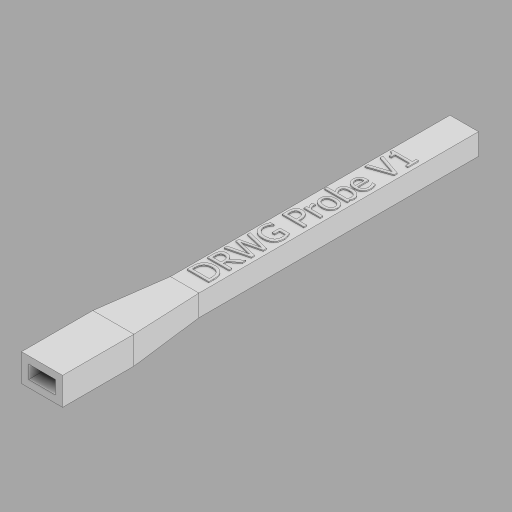
# Autodesk Inventor part: DRWG_ProbeAntenna_V1
Saved by Autodesk Inventor 2023 (Build 270158000, 158)
## iProperties
Created: 2024-10-22
Part Number: DRWG_ProbeAntenna_V1
Material: Generisch
Document SubType Name: Modeling
Designer: Nils Bade
Density: 1 g/cm^3
Appearance: Vorgabe
Author: Nils Bade
Autodesk Inventor part; units mm, degrees
ref_plane "YZ Plane" through (0, 0, 0) normal (1, 0, 0) x (0, 1, 0)
ref_plane "XZ Plane" through (0, 0, 0) normal (0, 1, 0) x (-1, 0, 0)
ref_plane "XY Plane" through (0, 0, 0) normal (0, 0, 1) x (1, 0, 0)
sketch "Skizze1" plane through (0, 0, 0) normal (0, 0, 1) x (1, 0, 0)
  line L0 (-1, 0.5) -> (1, 0.5)
  line L1 (1, 0.5) -> (1, -0.5)
  line L2 (1, -0.5) -> (-1, -0.5)
  line L3 (-1, -0.5) -> (-1, 0.5)
  line L4 (-1, 0.5) -> (1, -0.5) construction
  line L5 (1, 0.5) -> (-1, -0.5) construction
  line L6 (-0.35, 0.5) -> (0.35, 0.5)
  line L7 (0.35, 0.5) -> (0.35, 0.275)
  line L8 (0.35, 0.275) -> (-0.35, 0.275)
  line L9 (-0.35, 0.275) -> (-0.35, 0.5)
  line L10 (0, -2.1) -> (0, 2.1) construction
  line L11 (-2.8, 0) -> (2.8, 0) construction
  line L12 (-0.35, -0.5) -> (0.35, -0.5)
  line L13 (0.35, -0.5) -> (0.35, -0.275)
  line L14 (0.35, -0.275) -> (-0.35, -0.275)
  line L15 (-0.35, -0.275) -> (-0.35, -0.5)
  line L16 (2, 1.5) -> (-2, 1.5)
  line L17 (-2, 1.5) -> (-2, -1.5)
  line L18 (-2, -1.5) -> (2, -1.5)
  line L19 (2, -1.5) -> (2, 1.5)
  point P0 (0, 0)
  point P1 (0, 0.5)
  point P2 (0, 0.5)
  point P3 (0, -0.5)
  point P4 (0, -0.5)
  dimension "d0" = 2
  dimension "d1" = 1
  dimension "d2" = 0.7
  dimension "d3" = 0.55
  dimension "d4" = 1
  constraints: 36 end point, 6 parallel, 6 symmetric about line, 4 midpoint, 3 perpendicular, 3 point on line, 2 horizontal, 3 other
  measures "d0" distance of L1.end L2.end
  measures "d1" distance of L0.end L1.end
  measures "d2" distance of L7.end L8.end
  measures "d3" distance between parallel lines of L8 L14
  measures "d4" distance between parallel lines of L0 L16
extrude "Extrusion1" add sketch "Skizze1" along normal blind 50 contours L0 L7 L8 L9 | L15 L14 L13 L2 | L19 L18 L17 L16
sketch "Skizze2" plane through (0, 0, 0) normal (0, 0, 1) x (1, 0, 0)
  line L0 (1.8795, 0.94) -> (-1.8795, 0.94)
  line L1 (-1.8795, 0.94) -> (-1.8795, -0.94)
  line L2 (-1.8795, -0.94) -> (1.8795, -0.94)
  line L3 (1.8795, -0.94) -> (1.8795, 0.94)
  line L4 (1.8795, 0.94) -> (-1.8795, -0.94) construction
  line L5 (-1.8795, 0.94) -> (1.8795, -0.94) construction
  line L6 (-2.8795, 1.94) -> (2.8795, 1.94)
  line L7 (2.8795, 1.94) -> (2.8795, -1.94)
  line L8 (2.8795, -1.94) -> (-2.8795, -1.94)
  line L9 (-2.8795, -1.94) -> (-2.8795, 1.94)
  point P0 (0, 0)
  dimension "d7" = 3.759
  dimension "d8" = 1.88
  dimension "d9" = 1
  constraints: 20 end point, 4 parallel, 2 midpoint, 2 perpendicular, 1 horizontal, 3 other
  measures "d7" distance of L1.end L2.end
  measures "d8" distance of L0.end L1.end
  measures "d9" distance between parallel lines of L0 L6
extrude "Extrusion2" add sketch "Skizze2" along normal blind 10 from surface at 50
chamfer "Fase1-Taper" distance 0.879 distance2 20 1 edges at (-1, 0, 50) measured on face at (-1.5, 0, 50)
chamfer "Fase2-Taper" distance 0.879 distance2 20 1 edges at (1, 0, 50) measured on face at (1.5, 0, 50)
chamfer "Fase3-Taper" distance 0.44 distance2 20 4 edges at (1.4395, -0.5, 50) (0.675, -0.5, 50) (-0.675, -0.5, 50) (-1.4395, -0.5, 50) measured on face at (1.4395, -0.6, 50) measured on face at (-0.675, -0.6, 50) measured on face at (0.675, -0.6, 50) measured on face at (-1.4395, -0.6, 50)
chamfer "Fase4-Taper" distance 0.44 distance2 20 2 edges at (-1.4395, 0.5, 50) (-0.675, 0.5, 50) measured on face at (-1.4395, 0.6, 50) measured on face at (-0.675, 0.6, 50)
chamfer "Fase5-Taper" distance 0.44 distance2 20 2 edges at (0.675, 0.5, 50) (1.4395, 0.5, 50) measured on face at (0.675, 0.6, 50) measured on face at (1.4395, 0.6, 50)
chamfer "Fase7-Taper" distance 0.665 distance2 20 1 edges at (0, 0.275, 50) measured on face at (0, 0.775, 50)
chamfer "Fase8-Taper" distance 0.665 distance2 20 1 edges at (0, -0.275, 50) measured on face at (0, -0.775, 50)
chamfer "Fase9" distance 0.8 angle 45 4 edges at (0, 1.5, 0) (2, 0, 0) (0, -1.5, 0) (-2, 0, 0)
chamfer "Fase10" [suppressed]
chamfer "Fase11" distance 0.44 distance2 10 1 edges at (0, 1.5, 50) measured on face at (0, 1.6, 50)
chamfer "Fase12" distance 0.44 distance2 10 1 edges at (0, -1.5, 50) measured on face at (0, -1.6, 50)
chamfer "Fase13" distance 0.879 distance2 10 3 edges at (2, -1.72, 50) (2, 0, 50) (2, 1.72, 50) measured on face at (2.5, 1.72, 50) measured on face at (2.5, 0, 50) measured on face at (2.5, -1.72, 50)
chamfer "Fase14" distance 0.879 distance2 10 3 edges at (-2, -1.72, 50) (-2, 0, 50) (-2, 1.72, 50) measured on face at (-2.5, 0, 50) measured on face at (-2.5, -1.72, 50) measured on face at (-2.5, 1.72, 50)
ref_plane "CutSimEnde" through (0, 0, 10) normal (0, 0, -1) x (-1, 0, 0)
feature "Trennen1" [suppressed]
sketch "Skizze3" plane through (-2, 1.5, 0.8) normal (0, 1, 0) x (1, 0, 0)
  line L0 (0.2777, -37.5866) -> (0.2777, -7.5364) construction
  line L1 (0.2777, -7.5364) -> (3.5258, -7.5364) construction
  line L2 (3.5258, -7.5364) -> (3.5258, -37.5866) construction
  line L3 (3.5258, -37.5866) -> (0.2777, -37.5866) construction
  spline S0 degree 2 poles (1.9401, -34.8746) (2.3575, -34.8746) (3.0293, -35.213) (3.2171, -35.497) knots 0 0 0 1 2 2 2
  spline S1 degree 2 poles (3.2171, -35.497) (3.3628, -35.7292) (3.4616, -36.2059) (3.4616, -36.5764) knots 0 0 0 1 2 2 2
  line L4 (3.4616, -36.5764) -> (3.4616, -37.2779)
  line L5 (3.4616, -37.2779) -> (0.4136, -37.2779)
  line L6 (0.4136, -37.2779) -> (0.4136, -36.5838)
  spline S2 degree 2 poles (0.4136, -36.5838) (0.4136, -36.154) (0.542, -35.665) (0.6557, -35.4921) knots 0 0 0 1 2 2 2
  spline S3 degree 2 poles (0.6557, -35.4921) (0.8508, -35.1981) (1.4955, -34.8746) (1.9401, -34.8746) knots 0 0 0 1 2 2 2
  spline S4 degree 2 poles (1.9351, -35.2969) (1.5844, -35.2969) (1.0879, -35.5291) (0.9471, -35.7588) knots 0 0 0 1 2 2 2
  spline S5 degree 2 poles (0.9471, -35.7588) (0.8508, -35.9219) (0.7643, -36.2899) (0.7643, -36.5641) knots 0 0 0 1 2 2 2
  line L7 (0.7643, -36.5641) -> (0.7643, -36.8728)
  line L8 (0.7643, -36.8728) -> (3.1109, -36.8728)
  line L9 (3.1109, -36.8728) -> (3.1109, -36.5641)
  spline S6 degree 2 poles (3.1109, -36.5641) (3.1109, -36.2948) (3.0244, -35.8873) (2.9083, -35.7218) knots 0 0 0 1 2 2 2
  spline S7 degree 2 poles (2.9083, -35.7218) (2.765, -35.5094) (2.2908, -35.2969) (1.9351, -35.2969) knots 0 0 0 1 2 2 2
  line L10 (3.4616, -32.076) -> (3.4616, -32.6022)
  line L11 (3.4616, -32.6022) -> (2.2488, -33.5655)
  line L12 (2.2488, -33.5655) -> (2.2488, -34.0298)
  line L13 (2.2488, -34.0298) -> (3.4616, -34.0298)
  line L14 (3.4616, -34.0298) -> (3.4616, -34.4349)
  line L15 (3.4616, -34.4349) -> (0.4136, -34.4349)
  line L16 (0.4136, -34.4349) -> (0.4136, -33.6494)
  spline S8 degree 2 poles (0.4136, -33.6494) (0.4136, -33.3876) (0.4704, -33.0344) (0.5741, -32.8739) knots 0 0 0 1 2 2 2
  spline S9 degree 2 poles (0.5741, -32.8739) (0.6779, -32.7133) (1.0015, -32.5281) (1.241, -32.5281) knots 0 0 0 1 2 2 2
  spline S10 degree 2 poles (1.241, -32.5281) (1.5745, -32.5281) (2.0265, -32.8689) (2.1352, -33.1604) knots 0 0 0 1 2 2 2
  line L17 (2.1352, -33.1604) -> (3.4616, -32.076)
  spline S11 degree 2 poles (1.2732, -32.9504) (1.1398, -32.9504) (0.9348, -33.0443) (0.8681, -33.1431) knots 0 0 0 1 2 2 2
  spline S12 degree 2 poles (0.8681, -33.1431) (0.8113, -33.2295) (0.7643, -33.4593) (0.7643, -33.6272) knots 0 0 0 1 2 2 2
  line L18 (0.7643, -33.6272) -> (0.7643, -34.0298)
  line L19 (0.7643, -34.0298) -> (1.9104, -34.0298)
  line L20 (1.9104, -34.0298) -> (1.9104, -33.6741)
  spline S13 degree 2 poles (1.9104, -33.6741) (1.9104, -33.4988) (1.8487, -33.2197) (1.7523, -33.1233) knots 0 0 0 1 2 2 2
  spline S14 degree 2 poles (1.7523, -33.1233) (1.6684, -33.0344) (1.4312, -32.9504) (1.2732, -32.9504) knots 0 0 0 1 2 2 2
  line L21 (0.4136, -28.4179) -> (3.4616, -29.1837)
  line L22 (3.4616, -29.1837) -> (3.4616, -29.6381)
  line L23 (3.4616, -29.6381) -> (0.9323, -30.2581)
  line L24 (0.9323, -30.2581) -> (3.4616, -30.8608)
  line L25 (3.4616, -30.8608) -> (3.4616, -31.3103)
  line L26 (3.4616, -31.3103) -> (0.4136, -32.0884)
  line L27 (0.4136, -32.0884) -> (0.4136, -31.671)
  line L28 (0.4136, -31.671) -> (2.9404, -31.0584)
  line L29 (2.9404, -31.0584) -> (0.4136, -30.4508)
  line L30 (0.4136, -30.4508) -> (0.4136, -30.0383)
  line L31 (0.4136, -30.0383) -> (2.9701, -29.4257)
  line L32 (2.9701, -29.4257) -> (0.4136, -28.8156)
  line L33 (0.4136, -28.8156) -> (0.4136, -28.4179)
  spline S15 degree 2 poles (3.5209, -26.7779) (3.5209, -27.1014) (3.3233, -27.6374) (3.1232, -27.8301) knots 0 0 0 1 2 2 2
  spline S16 degree 2 poles (3.1232, -27.8301) (2.9207, -28.0227) (2.3229, -28.2278) (1.9351, -28.2278) knots 0 0 0 1 2 2 2
  spline S17 degree 2 poles (1.9351, -28.2278) (1.5671, -28.2278) (0.9842, -28.0203) (0.7767, -27.8276) knots 0 0 0 1 2 2 2
  spline S18 degree 2 poles (0.7767, -27.8276) (0.5766, -27.6424) (0.3593, -27.099) (0.3593, -26.7754) knots 0 0 0 1 2 2 2
  spline S19 degree 2 poles (0.3593, -26.7754) (0.3593, -26.6198) (0.4037, -26.3382) (0.4432, -26.2098) knots 0 0 0 1 2 2 2
  spline S20 degree 2 poles (0.4432, -26.2098) (0.4729, -26.106) (0.5816, -25.8541) (0.6211, -25.7775) knots 0 0 0 1 2 2 2
  line L34 (0.6211, -25.7775) -> (1.1101, -25.7775)
  line L35 (1.1101, -25.7775) -> (1.1101, -25.8121)
  spline S21 degree 2 poles (1.1101, -25.8121) (1.0434, -25.8887) (0.9224, -26.0492) (0.8533, -26.1974) knots 0 0 0 1 2 2 2
  spline S22 degree 2 poles (0.8533, -26.1974) (0.7915, -26.3209) (0.71, -26.6395) (0.71, -26.8223) knots 0 0 0 1 2 2 2
  spline S23 degree 2 poles (0.71, -26.8223) (0.71, -27.262) (1.372, -27.8054) (1.9228, -27.8054) knots 0 0 0 1 2 2 2
  spline S24 degree 2 poles (1.9228, -27.8054) (2.2291, -27.8054) (2.6885, -27.6621) (2.8466, -27.5263) knots 0 0 0 1 2 2 2
  spline S25 degree 2 poles (2.8466, -27.5263) (3.0046, -27.3954) (3.1701, -27.0249) (3.1701, -26.7927) knots 0 0 0 1 2 2 2
  spline S26 degree 2 poles (3.1701, -26.7927) (3.1701, -26.6222) (3.1207, -26.2814) (3.0713, -26.1653) knots 0 0 0 1 2 2 2
  line L36 (3.0713, -26.1653) -> (2.2834, -26.1653)
  line L37 (2.2834, -26.1653) -> (2.2834, -26.8717)
  line L38 (2.2834, -26.8717) -> (1.9277, -26.8717)
  line L39 (1.9277, -26.8717) -> (1.9277, -25.7652)
  line L40 (1.9277, -25.7652) -> (3.2591, -25.7652)
  spline S27 degree 2 poles (3.2591, -25.7652) (3.2936, -25.8417) (3.3998, -26.1035) (3.432, -26.2147) knots 0 0 0 1 2 2 2
  spline S28 degree 2 poles (3.432, -26.2147) (3.4764, -26.3654) (3.5209, -26.6074) (3.5209, -26.7779) knots 0 0 0 1 2 2 2
  spline S29 degree 2 poles (1.3324, -22.0206) (1.53, -22.0206) (1.8857, -22.1614) (2.0092, -22.2874) knots 0 0 0 1 2 2 2
  spline S30 degree 2 poles (2.0092, -22.2874) (2.1648, -22.4454) (2.3254, -22.8728) (2.3254, -23.1988) knots 0 0 0 1 2 2 2
  line L41 (2.3254, -23.1988) -> (2.3254, -23.5421)
  line L42 (2.3254, -23.5421) -> (3.4616, -23.5421)
  line L43 (3.4616, -23.5421) -> (3.4616, -23.9472)
  line L44 (3.4616, -23.9472) -> (0.4136, -23.9472)
  line L45 (0.4136, -23.9472) -> (0.4136, -23.1815)
  spline S31 degree 2 poles (0.4136, -23.1815) (0.4136, -22.9098) (0.5025, -22.5294) (0.6038, -22.3837) knots 0 0 0 1 2 2 2
  spline S32 degree 2 poles (0.6038, -22.3837) (0.7199, -22.2133) (1.078, -22.0206) (1.3324, -22.0206) knots 0 0 0 1 2 2 2
  spline S33 degree 2 poles (1.3448, -22.443) (1.1867, -22.443) (0.9545, -22.5517) (0.8804, -22.6628) knots 0 0 0 1 2 2 2
  spline S34 degree 2 poles (0.8804, -22.6628) (0.8162, -22.7591) (0.7643, -23.016) (0.7643, -23.2062) knots 0 0 0 1 2 2 2
  line L46 (0.7643, -23.2062) -> (0.7643, -23.5421)
  line L47 (0.7643, -23.5421) -> (1.9796, -23.5421)
  line L48 (1.9796, -23.5421) -> (1.9796, -23.2655)
  spline S35 degree 2 poles (1.9796, -23.2655) (1.9796, -23.0185) (1.9005, -22.7147) (1.7968, -22.6159) knots 0 0 0 1 2 2 2
  spline S36 degree 2 poles (1.7968, -22.6159) (1.7054, -22.5245) (1.4905, -22.443) (1.3448, -22.443) knots 0 0 0 1 2 2 2
  line L49 (1.5869, -20.4521) -> (1.5869, -20.4719)
  spline S37 degree 2 poles (1.5869, -20.4719) (1.5745, -20.5164) (1.5696, -20.6127) (1.5696, -20.6794) knots 0 0 0 1 2 2 2
  spline S38 degree 2 poles (1.5696, -20.6794) (1.5696, -20.835) (1.7054, -21.1413) (1.8388, -21.2796) knots 0 0 0 1 2 2 2
  line L50 (1.8388, -21.2796) -> (3.4616, -21.2796)
  line L51 (3.4616, -21.2796) -> (3.4616, -21.6649)
  line L52 (3.4616, -21.6649) -> (1.1744, -21.6649)
  line L53 (1.1744, -21.6649) -> (1.1744, -21.2796)
  line L54 (1.1744, -21.2796) -> (1.5152, -21.2796)
  spline S39 degree 2 poles (1.5152, -21.2796) (1.3275, -21.0696) (1.1744, -20.756) (1.1744, -20.6078) knots 0 0 0 1 2 2 2
  spline S40 degree 2 poles (1.1744, -20.6078) (1.1744, -20.5485) (1.1793, -20.4892) (1.1867, -20.4521) knots 0 0 0 1 2 2 2
  line L55 (1.1867, -20.4521) -> (1.5869, -20.4521)
  spline S41 degree 2 poles (2.318, -18.2736) (2.896, -18.2736) (3.5258, -18.8293) (3.5258, -19.2937) knots 0 0 0 1 2 2 2
  spline S42 degree 2 poles (3.5258, -19.2937) (3.5258, -19.7704) (2.8762, -20.3163) (2.318, -20.3163) knots 0 0 0 1 2 2 2
  spline S43 degree 2 poles (2.318, -20.3163) (1.7449, -20.3163) (1.1101, -19.7531) (1.1101, -19.2937) knots 0 0 0 1 2 2 2
  spline S44 degree 2 poles (1.1101, -19.2937) (1.1101, -18.8293) (1.7425, -18.2736) (2.318, -18.2736) knots 0 0 0 1 2 2 2
  spline S45 degree 2 poles (2.318, -18.6713) (1.8734, -18.6713) (1.4411, -18.9948) (1.4411, -19.2937) knots 0 0 0 1 2 2 2
  spline S46 degree 2 poles (1.4411, -19.2937) (1.4411, -19.5926) (1.8734, -19.9186) (2.318, -19.9186) knots 0 0 0 1 2 2 2
  spline S47 degree 2 poles (2.318, -19.9186) (2.7502, -19.9186) (3.1948, -19.5926) (3.1948, -19.2937) knots 0 0 0 1 2 2 2
  spline S48 degree 2 poles (3.1948, -19.2937) (3.1948, -18.9973) (2.7576, -18.6713) (2.318, -18.6713) knots 0 0 0 1 2 2 2
  spline S49 degree 2 poles (2.2809, -15.9617) (2.8416, -15.9617) (3.5258, -16.5051) (3.5258, -16.9151) knots 0 0 0 1 2 2 2
  spline S50 degree 2 poles (3.5258, -16.9151) (3.5258, -17.1003) (3.4344, -17.3646) (3.3554, -17.4931) knots 0 0 0 1 2 2 2
  line L56 (3.3554, -17.4931) -> (3.4616, -17.5178)
  line L57 (3.4616, -17.5178) -> (3.4616, -17.8784)
  line L58 (3.4616, -17.8784) -> (0.2777, -17.8784)
  line L59 (0.2777, -17.8784) -> (0.2777, -17.4931)
  line L60 (0.2777, -17.4931) -> (1.4139, -17.4931)
  spline S51 degree 2 poles (1.4139, -17.4931) (1.283, -17.3473) (1.1101, -17.0089) (1.1101, -16.7941) knots 0 0 0 1 2 2 2
  spline S52 degree 2 poles (1.1101, -16.7941) (1.1101, -16.4063) (1.7301, -15.9617) (2.2809, -15.9617) knots 0 0 0 1 2 2 2
  spline S53 degree 2 poles (2.3106, -16.3593) (1.9005, -16.3593) (1.4757, -16.6088) (1.4757, -16.8854) knots 0 0 0 1 2 2 2
  spline S54 degree 2 poles (1.4757, -16.8854) (1.4757, -17.0411) (1.6239, -17.3622) (1.7375, -17.4931) knots 0 0 0 1 2 2 2
  line L61 (1.7375, -17.4931) -> (3.0491, -17.4931)
  spline S55 degree 2 poles (3.0491, -17.4931) (3.1207, -17.3473) (3.18, -17.1226) (3.18, -16.9892) knots 0 0 0 1 2 2 2
  spline S56 degree 2 poles (3.18, -16.9892) (3.18, -16.6953) (2.7626, -16.3593) (2.3106, -16.3593) knots 0 0 0 1 2 2 2
  spline S57 degree 2 poles (3.5135, -14.5686) (3.5135, -15.1169) (2.8984, -15.7196) (2.3303, -15.7196) knots 0 0 0 1 2 2 2
  spline S58 degree 2 poles (2.3303, -15.7196) (1.7721, -15.7196) (1.1101, -15.1342) (1.1101, -14.6624) knots 0 0 0 1 2 2 2
  spline S59 degree 2 poles (1.1101, -14.6624) (1.1101, -14.45) (1.2336, -14.1215) (1.3645, -14.0005) knots 0 0 0 1 2 2 2
  spline S60 degree 2 poles (1.3645, -14.0005) (1.4955, -13.877) (1.8734, -13.7461) (2.1475, -13.7461) knots 0 0 0 1 2 2 2
  line L62 (2.1475, -13.7461) -> (2.3575, -13.7461)
  line L63 (2.3575, -13.7461) -> (2.3575, -15.3293)
  spline S61 degree 2 poles (2.3575, -15.3293) (2.7552, -15.3293) (3.1775, -14.9292) (3.1775, -14.5735) knots 0 0 0 1 2 2 2
  spline S62 degree 2 poles (3.1775, -14.5735) (3.1775, -14.4475) (3.1207, -14.203) (3.0763, -14.1042) knots 0 0 0 1 2 2 2
  spline S63 degree 2 poles (3.0763, -14.1042) (3.0269, -14.0005) (2.9404, -13.8572) (2.9009, -13.8103) knots 0 0 0 1 2 2 2
  line L64 (2.9009, -13.8103) -> (2.9009, -13.788)
  line L65 (2.9009, -13.788) -> (3.3208, -13.788)
  spline S64 degree 2 poles (3.3208, -13.788) (3.348, -13.8547) (3.427, -14.0573) (3.4492, -14.1363) knots 0 0 0 1 2 2 2
  spline S65 degree 2 poles (3.4492, -14.1363) (3.4814, -14.2475) (3.5135, -14.4302) (3.5135, -14.5686) knots 0 0 0 1 2 2 2
  spline S66 degree 2 poles (2.0636, -14.1215) (1.908, -14.1264) (1.6807, -14.1907) (1.6041, -14.2524) knots 0 0 0 1 2 2 2
  spline S67 degree 2 poles (1.6041, -14.2524) (1.5177, -14.3191) (1.4263, -14.529) (1.4263, -14.6847) knots 0 0 0 1 2 2 2
  spline S68 degree 2 poles (1.4263, -14.6847) (1.4263, -14.8378) (1.5177, -15.0527) (1.6066, -15.1416) knots 0 0 0 1 2 2 2
  spline S69 degree 2 poles (1.6066, -15.1416) (1.698, -15.2281) (1.9178, -15.317) (2.0636, -15.3293) knots 0 0 0 1 2 2 2
  line L66 (2.0636, -15.3293) -> (2.0636, -14.1215)
  line L67 (0.4136, -9.8064) -> (3.4616, -10.8561)
  line L68 (3.4616, -10.8561) -> (3.4616, -11.2933)
  line L69 (3.4616, -11.2933) -> (0.4136, -12.3431)
  line L70 (0.4136, -12.3431) -> (0.4136, -11.9084)
  line L71 (0.4136, -11.9084) -> (2.9454, -11.0636)
  line L72 (2.9454, -11.0636) -> (0.4136, -10.2189)
  line L73 (0.4136, -10.2189) -> (0.4136, -9.8064)
  line L74 (3.4616, -7.8748) -> (3.4616, -9.3618)
  line L75 (3.4616, -9.3618) -> (3.1504, -9.3618)
  line L76 (3.1504, -9.3618) -> (3.1504, -8.8085)
  line L77 (3.1504, -8.8085) -> (1.1077, -8.8085)
  line L78 (1.1077, -8.8085) -> (1.1077, -9.3618)
  line L79 (1.1077, -9.3618) -> (0.8286, -9.3618)
  spline S70 degree 2 poles (0.8286, -9.3618) (0.8286, -9.0481) (0.6507, -8.7517) (0.4037, -8.7319) knots 0 0 0 1 2 2 2
  line L80 (0.4037, -8.7319) -> (0.4037, -8.4158)
  line L81 (0.4037, -8.4158) -> (3.1504, -8.4158)
  line L82 (3.1504, -8.4158) -> (3.1504, -7.8748)
  line L83 (3.1504, -7.8748) -> (3.4616, -7.8748)
  point P0 (2, 0.8)
  constraints: 2 other
extrude "Extrusion3" add sketch "Skizze3" along normal blind 0.15
equation "\"d13\" = Taperlänge"
equation "\"d16\" = Taperlänge"
equation "\"d19\" = Taperlänge"
equation "\"d22\" = Taperlänge"
equation "\"d25\" = Taperlänge"
equation "\"d31\" = Taperlänge"
equation "\"d34\" = Taperlänge"
equation "\"Taperlänge\" = 20"
